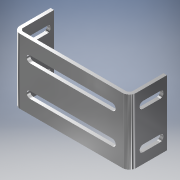
# Autodesk Inventor part: thumbkey_cup
Saved by Autodesk Inventor 2018 (Build 220112000, 112)
## iProperties
Created: 2018-04-06
Part Number: thumbkey_cup
Material: アルミニウム 6061
Document SubType Name: Sheet Metal
Designer: NaMACHAN
Density: 2.7 g/cm^3
Sheet Metal Rule: Default_mm
Appearance: アルミニウム - フラット
Mass: 27.9111 g
Surface Area: 87.5065 cm^2
Volume: 10.3374 cm^3
Author: NaMACHAN
Autodesk Inventor part; units mm, degrees
ref_plane "YZ Plane" through (0, 0, 0) normal (1, 0, 0) x (0, 1, 0)
ref_plane "XZ Plane" through (0, 0, 0) normal (0, 1, 0) x (-1, 0, 0)
ref_plane "XY Plane" through (0, 0, 0) normal (0, 0, 1) x (1, 0, 0)
sketch "スケッチ1" plane through (0, 0, 0) normal (0, 1, 0) x (-1, 0, 0)
  line L0 (-32, -19) -> (32, -19)
  line L1 (32, -19) -> (32, 19)
  line L2 (32, 19) -> (-32, 19)
  line L3 (-32, 19) -> (-32, -19)
  line L4 (-32, -19) -> (32, 19) construction
  line L5 (32, -19) -> (-32, 19) construction
  point P0 (0, 0)
  dimension "d0" = 38
  dimension "d1" = 64
  measures "d0" distance of L0.end L1.end
  measures "d1" distance of L0.start L0.end
extrude "プレート1" add sketch "スケッチ1" along normal blind 2
sketch "スケッチ2" plane through (32, 0, 19) normal (1, 0, 0) x (0, 0, -1)
  line L0 (0, 2) -> (38, 2)
  line L1 (38, 2) -> (0, 2)
  line L2 (0, 2) -> (0, 22)
  line L3 (0, 22) -> (38, 22)
  line L4 (38, 22) -> (38, 2)
  point P0 (19, 0)
  dimension "d3" = 20
  measures "d3" distance of L3.end L0.end
sheet face with bend "面2" sketch "スケッチ2" thickness 2 toward (1, 0, 0) bend radius 2 relief straight relief width 2 relief depth 1
bend "曲げ1"
sketch "スケッチ3" plane through (-32, 0, -19) normal (-1, 0, 0) x (0, 0, 1)
  line L0 (0, 0) -> (0, 2)
  line L1 (0, 22) -> (38, 22)
  line L2 (0, 2) -> (38, 2)
  line L3 (38, 2) -> (38, 22)
  line L4 (38, 22) -> (0, 22)
  line L5 (0, 22) -> (0, 2)
  point P0 (19, 0)
sheet face with bend "面3" sketch "スケッチ3" thickness 2 toward (-1, 0, 0) bend radius 2 relief straight relief width 2 relief depth 1
bend "曲げ2"
sketch "スケッチ4" plane through (-34, 0, -19) normal (-1, 0, 0) x (0, 0, 1)
  line L0 (6, 18) -> (6, 8)
  arc A0 (6, 8) -> (10, 8) centre (8, 8) ccw
  line L1 (10, 8) -> (10, 18)
  arc A1 (10, 18) -> (6, 18) centre (8, 18) ccw
  line L2 (0, 22) -> (38, 22) projected
  line L3 (38, 4) -> (0, 4) projected
  line L4 (0, 4) -> (0, 22) projected
  line L5 (28, 18) -> (28, 8)
  arc A2 (28, 8) -> (32, 8) centre (30, 8) ccw
  line L6 (32, 8) -> (32, 18)
  arc A3 (32, 18) -> (28, 18) centre (30, 18) ccw
  line L7 (38, 22) -> (38, 4) projected
  point P0 (19, 0)
  dimension "d14" = 2
  dimension "d15" = 4
  dimension "d16" = 4
  dimension "d17" = 6
  dimension "d18" = 2
  dimension "d19" = 6
  constraints: 8 end point, 8 point on circle, 8 tangent, 4 centre point, 2 horizontal alignment, 2 parallel, 2 vertical
  measures "d14" radius of A1
  measures "d15" distance from line of L2 A1.centre
  measures "d16" distance from line of L3 A0.centre
  measures "d17" distance between parallel lines of L4 L0
  measures "d18" radius of A3
  measures "d19" distance between parallel lines of L7 L6
extrude "押し出し1" cut sketch "スケッチ4" against normal blind 100 contours A1 L1 A0 L0 | A3 L6 A2 L5
sketch "スケッチ5" plane through (0, 2, 0) normal (0, 1, 0) x (1, 0, 0)
  line L0 (-24, -11) -> (24, -11)
  arc A0 (24, -11) -> (24, -7) centre (24, -9) ccw
  line L1 (24, -7) -> (-24, -7)
  arc A1 (-24, -7) -> (-24, -11) centre (-24, -9) ccw
  line L2 (-24, 7) -> (24, 7)
  arc A2 (24, 7) -> (24, 11) centre (24, 9) ccw
  line L3 (24, 11) -> (-24, 11)
  arc A3 (-24, 11) -> (-24, 7) centre (-24, 9) ccw
  line L4 (-30, 19) -> (30, 19) projected
  line L5 (30, -19) -> (-30, -19) projected
  line L6 (-30, 19) -> (-30, -19) projected
  line L7 (30, -19) -> (30, 19) projected
  point P0 (0, 0)
  dimension "d22" = 2
  dimension "d23" = 2
  dimension "d25" = 10
  dimension "d26" = 10
  dimension "d27" = 6
  dimension "d28" = 6
  dimension "d29" = 6
  dimension "d30" = 6
  constraints: 8 end point, 8 point on circle, 8 tangent, 4 centre point, 2 horizontal, 2 parallel
  measures "d22" radius of A1
  measures "d23" radius of A3
  measures "d25" distance from line of L4 A3.centre
  measures "d26" distance from line of L5 A1.centre
  measures "d27" distance from line of L6 A1.centre
  measures "d28" distance from line of L6 A3.centre
  measures "d29" distance from line of L7 A2.centre
  measures "d30" distance from line of L7 A0.centre
extrude "押し出し2" cut sketch "スケッチ5" against normal blind 3 contours A1 L1 A0 L0 | A3 L3 A2 L2
equation "\"d2\" = Thickness"
equation "\"d4\" = BendRadius"
equation "\"d5\" = BendReliefWidth"
equation "\"d7\" = MinimumRemnant"
equation "\"d6\" = BendReliefDepth"
equation "\"d8\" = TransitionRadius"
equation "\"d9\" = BendRadius"
equation "\"d10\" = BendReliefWidth"
equation "\"d12\" = MinimumRemnant"
equation "\"d11\" = BendReliefDepth"
equation "\"d13\" = TransitionRadius"
equation "\"BendRadius\" = Thickness"
equation "\"BendReliefWidth\" = Thickness"
equation "\"BendReliefDepth\" = 0.5 * Thickness"
equation "\"CornerReliefSize\" = 4 * Thickness"
equation "\"MinimumRemnant\" = 2 * Thickness"
equation "\"TransitionRadius\" = BendRadius"
equation "\"JacobiRadiusSize\" = BendRadius"
equation "\"GapSize\" = Thickness"
equation "\"Thickness\" = 2"
